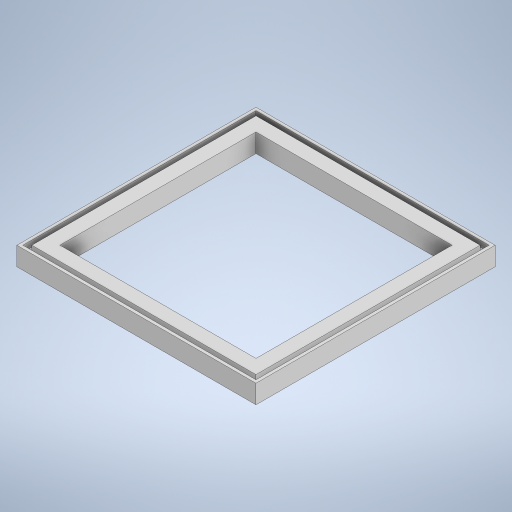
# Autodesk Inventor part: 사각형 OV-PAM 5패턴 링
Saved by Autodesk Inventor 2024 (Build 280153000, 153)
## iProperties
Created: 2023-06-19
Part Number: 사각형 OV-PAM 5패턴 링
Material: 일반
Document SubType Name: Modeling
Designer: jsw
Density: 1 g/cm^3
Appearance: 기본값
Author: jsw
Autodesk Inventor part; units mm, degrees
ref_plane "YZ Plane" through (0, 0, 0) normal (1, 0, 0) x (0, 1, 0)
ref_plane "XZ Plane" through (0, 0, 0) normal (0, 1, 0) x (-1, 0, 0)
ref_plane "XY Plane" through (0, 0, 0) normal (0, 0, 1) x (1, 0, 0)
sketch "스케치1" plane through (0, 0, 0) normal (0, 1, 0) x (-1, 0, 0)
  line L0 (-32, -32) -> (32, -32)
  line L1 (32, -32) -> (32, 32)
  line L2 (32, 32) -> (-32, 32)
  line L3 (-32, 32) -> (-32, -32)
  line L4 (-32, -32) -> (32, 32) construction
  line L5 (32, -32) -> (-32, 32) construction
  point P0 (0, 0)
  dimension "d0" = 64
  dimension "d1" = 64
  constraints: 12 end point, 2 midpoint, 2 parallel, 1 horizontal, 1 perpendicular
  measures "d0" distance of L2.end L1.end
  measures "d1" distance of L1.end L0.end
extrude "돌출1" add sketch "스케치1" along normal blind 5
sketch "스케치2" plane through (0, 5, 0) normal (0, 1, 0) x (1, 0, 0)
  line L0 (30, 30) -> (-30, 30)
  line L1 (-30, 30) -> (-30, -30)
  line L2 (-30, -30) -> (30, -30)
  line L3 (30, -30) -> (30, 30)
  line L4 (30, 30) -> (-30, -30) construction
  line L5 (-30, 30) -> (30, -30) construction
  line L6 (31.2, -31.2) -> (-31.2, -31.2)
  line L7 (-31.2, -31.2) -> (-31.2, 31.2)
  line L8 (-31.2, 31.2) -> (31.2, 31.2)
  line L9 (31.2, 31.2) -> (31.2, -31.2)
  line L10 (31.2, -31.2) -> (-31.2, 31.2) construction
  line L11 (-31.2, -31.2) -> (31.2, 31.2) construction
  point P0 (0, 0)
  dimension "d4" = 60
  dimension "d5" = 60
  dimension "d6" = 1.2
  constraints: 24 end point, 4 midpoint, 4 parallel, 2 horizontal, 2 perpendicular, 1 point on line
  measures "d4" distance of L0.end L1.end
  measures "d5" distance of L1.end L2.end
  measures "d6" distance between parallel lines of L2 L6
extrude "돌출2" cut sketch "스케치2" against normal blind 1.6
sketch "스케치3" plane through (0, 5, 0) normal (0, 1, 0) x (1, 0, 0)
  line L0 (26.25, -26.25) -> (-26.25, -26.25)
  line L1 (-26.25, -26.25) -> (-26.25, 26.25)
  line L2 (-26.25, 26.25) -> (26.25, 26.25)
  line L3 (26.25, 26.25) -> (26.25, -26.25)
  line L4 (26.25, -26.25) -> (-26.25, 26.25) construction
  line L5 (-26.25, -26.25) -> (26.25, 26.25) construction
  point P0 (0, 0)
  dimension "d9" = 52.5
  dimension "d10" = 52.5
  constraints: 12 end point, 2 midpoint, 2 parallel, 1 horizontal, 1 perpendicular
  measures "d9" distance of L0.end L1.end
  measures "d10" distance of L0.start L0.end
extrude "돌출3" cut sketch "스케치3" against normal blind 5
ref_plane "작업 평면1" through (0, 2.5, 0) normal (0, 1, 0) x (1, 0, 0)
mirror "미러1" about plane through (0, 2.5, 0) normal (0, 1, 0) of "돌출2"
